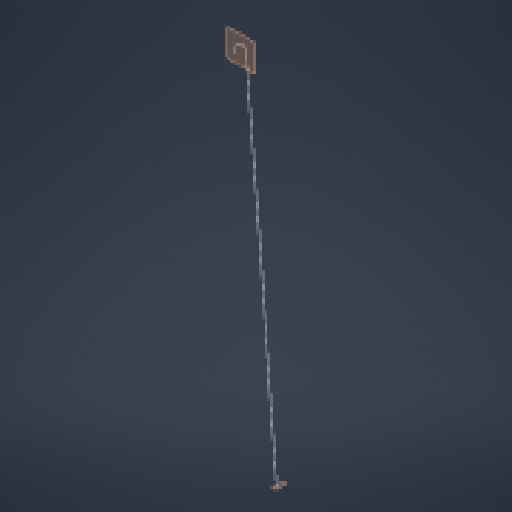
# Autodesk Inventor part: Ropes
Saved by Autodesk Inventor 2023.6 (Build 276521000, 521)
## iProperties
Created: 2026-03-05
Part Number: Ropes
Material: Generic
Document SubType Name: Modeling
Designer: user
Density: 1 g/cm^3
Appearance: Default
Author: user
Autodesk Inventor part; units mm, degrees
ref_plane "YZ Plane" through (0, 0, 0) normal (1, 0, 0) x (0, 1, 0)
ref_plane "XZ Plane" through (0, 0, 0) normal (0, 1, 0) x (-1, 0, 0)
ref_plane "XY Plane" through (0, 0, 0) normal (0, 0, 1) x (1, 0, 0)
ref_plane "Work Plane1" through (0, 0, 0) normal (0, 0, 1) x (1, 0, 0)
sketch "Sketch1" plane through (0, 0, 0) normal (0, 0, 1) x (1, 0, 0)
  circle A0 centre (0, 0) radius 5 projected
  line L0 (34.4218, -369.1091) -> (38.4068, -368.7629) projected
  arc A1 (5.4808, 0.459) -> (-5.5, 0) centre (0, 0) ccw
  line L1 (36.4143, -368.936) -> (5.4808, 0.459)
  line L2 (-5.5, 0) -> (-5.5, -5.5)
  point P0 (0, 0)
  dimension "d0" = 11
  constraints: 4 end point, 2 point on circle, 2 tangent, 1 centre point, 1 coincident, 1 midpoint, 1 vertical
  measures "d0" diameter of A1
ref_plane "Work Plane2" through (34.4218, -369.1091, -8) normal (-0.0865, 0.9962, 0) x (-0.9962, -0.0865, 0)
sketch "Sketch2" plane through (34.4218, -369.1091, -8) normal (-0.0865, 0.9962, 0) x (-0.9962, -0.0865, 0)
  circle A0 centre (-2, 8) radius 0.5
  point P0 (2.3507, 8)
  dimension "d1" = 1
  constraints: 1 centre point, 1 coincident
  measures "d1" diameter of A0
sweep "Sweep1" add profiles "Sketch2" path "Sketch1" path curves L1 A1 L2
body "Solid1"
